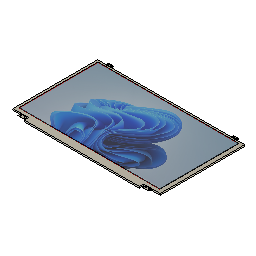
Panel_Enclosure (Autodesk Fusion 360 archive; units mm, degrees)
design "Panel_Physical"
Autodesk Fusion 360 part; units mm, degrees
sketch "Panel_Dims" plane through (0, 0, 0) normal (0, 0, 1) x (1, 0, 0)
  line L0 (-180, 103.5) -> (180, 103.5) construction
  line L1 (180, 103.5) -> (180, -103.5) construction
  line L2 (180, -103.5) -> (-180, -103.5) construction
  line L3 (-180, -103.5) -> (-180, 103.5) construction
  line L4 (0, 0) -> (0, 103.5) construction
  line L5 (0, 0) -> (-180, 0) construction
  line L6 (-160, -103.5) -> (-160, -111.5)
  line L7 (-145, -103.5) -> (-145, -111.5)
  line L8 (-145, -111.5) -> (-160, -111.5)
  line L9 (-142, -103.5) -> (-142, -114)
  line L10 (160, -103.5) -> (160, -111.5)
  line L11 (145, -103.5) -> (145, -111.5)
  line L12 (160, -111.5) -> (145, -111.5)
  line L13 (139.5, -103.5) -> (139.5, -114)
  line L14 (139.5, -114) -> (-142, -114)
  line L15 (-160, 103.5) -> (-160, 109.8)
  line L16 (-160, 109.8) -> (-147, 109.8)
  line L17 (-147, 109.8) -> (-147, 103.5)
  line L18 (160, 103.5) -> (160, 109.8)
  line L19 (160, 109.8) -> (147, 109.8)
  line L20 (147, 109.8) -> (147, 103.5)
  line L21 (-180, 103.5) -> (-180, -103.5)
  line L22 (-180, -103.5) -> (-160, -103.5)
  line L23 (-145, -103.5) -> (-142, -103.5)
  line L24 (145, -103.5) -> (139.5, -103.5)
  line L25 (160, -103.5) -> (180, -103.5)
  line L26 (180, 103.5) -> (180, -103.5)
  line L27 (-160, 103.5) -> (-180, 103.5)
  line L28 (-147, 103.5) -> (147, 103.5)
  line L29 (160, 103.5) -> (180, 103.5)
  line L30 (-142, -103.5) -> (139.5, -103.5)
  circle A0 centre (-156.5, -106.7) radius 1.2
  circle A1 centre (-148.5, -106.7) radius 1.2
  line L31 (-156.5, -106.7) -> (-148.5, -106.7) construction
  circle A2 centre (148.5, -106.7) radius 1.2
  line L32 (148.5, -106.7) -> (156.5, -106.7) construction
  circle A3 centre (156.5, -106.7) radius 1.2
  circle A4 centre (-156.5, 106.7) radius 1.2
  line L33 (-156.5, 106.7) -> (-150.5, 106.7) construction
  circle A5 centre (-150.5, 106.7) radius 1.2
  circle A6 centre (150.5, 106.7) radius 1.2
  line L34 (150.5, 106.7) -> (156.5, 106.7) construction
  circle A7 centre (156.5, 106.7) radius 1.2
  line L35 (-174.55, 99) -> (169.45, 99)
  line L36 (169.45, 99) -> (169.45, -94)
  line L37 (169.45, -94) -> (-174.55, -94)
  line L38 (-174.55, -94) -> (-174.55, 99)
  line L39 (145, -103.5) -> (160, -103.5)
  line L40 (147, 103.5) -> (160, 103.5)
  line L41 (-147, 103.5) -> (-160, 103.5)
  line L42 (-160, -103.5) -> (-145, -103.5)
  line L43 (-73, -103.5) -> (-43, -103.5)
  line L44 (-43, -103.5) -> (-43, -114)
  line L45 (-43, -114) -> (-73, -114)
  line L46 (-73, -114) -> (-73, -103.5)
  line L47 (-45, -105) -> (-70, -105)
  line L48 (-70, -105) -> (-70, -109)
  line L49 (-70, -109) -> (-45, -109)
  line L50 (-45, -109) -> (-45, -105)
  point P0 (-156.5, -106.7)
  dimension "panel_w" = 360
  dimension "panel_h" = 207
  dimension "ear_indent" = 20
  dimension "ear_bottom_w" = 15
  dimension "ear_bottom_h" = 8
  dimension "pcb_left_indent" = 38
  dimension "d37" = 20
  dimension "d40" = 8
  dimension "pcb_chin_h" = 10.5
  dimension "pcb_chin_w" = 281.5
  dimension "d45" = 20
  dimension "ear_top_h" = 6.3
  dimension "ear_top_w" = 13
  dimension "d48" = 20
  dimension "d49" = 6.3
  dimension "d50" = 13
  dimension "hole_dist_x" = 3.5
  dimension "hole_dia" = 2.4
  dimension "hole_dist_y" = 3.2
  dimension "d54" = 2.4
  dimension "hole_bottom_ipd" = 8
  dimension "d62" = 2.4
  dimension "d63" = 2.4
  dimension "d64" = 8
  dimension "d65" = 3.2
  dimension "d66" = 3.5
  dimension "d67" = 2.4
  dimension "d68" = 2.4
  dimension "hole_top_ipd" = 6
  dimension "d70" = 3.5
  dimension "d72" = 3.2
  dimension "d73" = 2.4
  dimension "d74" = 2.4
  dimension "d75" = 6
  dimension "d76" = 3.5
  dimension "d77" = 3.2
  dimension "bezel_left" = 5.45
  dimension "bezel_top" = 4.5
  dimension "active_w" = 344
  dimension "active_h" = 193
  dimension "d98" = 30
  dimension "d99" = 10.5
  dimension "d100" = 137
  dimension "d101" = 25
  dimension "d102" = 4
  dimension "d103" = 5
  dimension "d104" = 2
  constraint horizontal L0
  constraint vertical L1
  constraint horizontal L2
  constraint vertical L3
  constraint coincident L4.start L5.start
  constraint midpoint L0 L4.end
  constraint midpoint L3 L5.end
  constraint horizontal L5
  constraint vertical L4
  constraint coincident L2 L6.start
  constraint perpendicular L2 L6
  constraint coincident L2 L7.start
  constraint perpendicular L2 L7
  constraint coincident L2 L9.start
  constraint perpendicular L2 L9
  constraint coincident L2 L10.start
  constraint perpendicular L2 L10
  constraint equal L6 L7
  constraint coincident L2 L11.start
  constraint perpendicular L2 L11
  constraint equal L10 L11
  constraint equal L8 L12
  constraint coincident L2 L13.start
  constraint perpendicular L2 L13
  constraint equal L9 L13
  constraint perpendicular L9 L14
  constraint coincident L0 L15.start
  constraint perpendicular L0 L15
  constraint perpendicular L3 L16
  constraint coincident L0 L17.end
  constraint perpendicular L0 L17
  constraint coincident L0 L18.start
  constraint perpendicular L0 L18
  constraint perpendicular L18 L19
  constraint coincident L0 L20.end
  constraint perpendicular L0 L20
  constraint coincident P0 A0.centre
  constraint coincident A1.centre L31.end
  constraint horizontal L31
  constraint coincident A2.centre L32.start
  constraint coincident L32.end A3.centre
  constraint horizontal L32
  constraint coincident A4.centre L33.start
  constraint coincident L33.end A5.centre
  constraint horizontal L33
  constraint coincident A6.centre L34.start
  constraint coincident L34.end A7.centre
  constraint horizontal L34
  constraint horizontal L35
  constraint vertical L36
  constraint horizontal L37
  constraint vertical L38
  constraint horizontal L43
  constraint vertical L44
  constraint horizontal L45
  constraint vertical L46
  constraint coincident L30 L43.start
  constraint horizontal L47
  constraint vertical L48
  constraint horizontal L49
  constraint vertical L50
  measures "panel_w" distance of L1.end L2.end
  measures "panel_h" distance of L0.start L2.end
  measures "ear_indent" distance of L2.end L6.start
  measures "ear_bottom_w" distance of L6.start L7.start
  measures "ear_bottom_h" distance of L6.start L6.end
  measures "pcb_left_indent" distance of L2.end L9.start
  measures "d37" distance of L1.end L10
  measures "d40" distance of L10.start L10.end
  measures "pcb_chin_h" distance of L9.start L9.end
  measures "pcb_chin_w" distance of L9.end L13.end
  measures "d45" distance of L0.start L15.start
  measures "ear_top_h" distance of L15.start L15.end
  measures "ear_top_w" distance of L15.end L16.end
  measures "d48" distance of L0.end L18
  measures "d49" distance of L18.start L18.end
  measures "d50" distance of L18.end L19.end
  measures "hole_dist_x" horizontal distance of L6.start P0
  measures "hole_dia" diameter of A0
  measures "hole_dist_y" vertical distance of L6.start P0
  measures "d54" diameter of A1
  measures "hole_bottom_ipd" distance of P0 A1.centre
  measures "d62" diameter of A2
  measures "d63" diameter of A3
  measures "d64" distance of L32.end A2.centre
  measures "d65" distance of L2 L32.end
  measures "d66" distance of L10 L32.end
  measures "d67" diameter of A4
  measures "d68" diameter of A5
  measures "hole_top_ipd" distance of L33.end A4.centre
  measures "d70" distance of L15 A4.centre
  measures "d72" distance of L27 A4.centre
  measures "d73" diameter of A6
  measures "d74" diameter of A7
  measures "d75" distance of L34.end A6.centre
  measures "d76" distance of L18 L34.end
  measures "d77" distance of L0 L34.end
  measures "bezel_left" distance of L3 L38
  measures "bezel_top" distance of L27 L35
  measures "active_w" distance of L35.start L35.end
  measures "active_h" distance of L35.end L36.end
  measures "d98" distance of L43.start L43.end
  measures "d99" distance of L43.end L44.end
  measures "d100" distance of L21 L44
  measures "d101" distance of L47.start L47.end
  measures "d102" distance of L47.start L49.end
  measures "d103" distance of L14 L49
  measures "d104" distance of L44 L49.end
extrude "Extrude2" add sketch "Panel_Dims" against normal blind 3.8 from surface at 3.8 contours L9 L14 L30 L46 | L14 L30 L43 L44 L45 L46 | L13 L14 L30 L44 | L47 L48 L49 L50 makes body 1
extrude "Extrude4" add sketch "Panel_Dims" along normal blind 3 separate body contours L35 L36 L37 L38 makes body 2
extrude "Extrude5" add sketch "Panel_Dims" along normal blind 3.8 contours L21 L22 L23 L24 L25 L26 L27 L28 L29 L30 L39 L40 L41 L42 L43 bodies 1 2
extrude "Extrude6" add sketch "Panel_Dims" along normal blind 0.3 from surface at 3 contours L6 L7 L8 L42 | L15 L16 L17 L41 | L18 L19 L20 L40 | L10 L11 L12 L39 bodies 1
extrude "Extrude7" cut sketch "Panel_Dims" along normal blind 1 contours L47 L48 L49 L50 bodies 1
equation "d37 = ear_indent"
equation "d40 = ear_bottom_h"
equation "d45 = ear_indent"
equation "d48 = ear_indent"
equation "d49 = ear_top_h"
equation "d50 = ear_top_w"
equation "d54 = hole_dia"
equation "d62 = hole_dia"
equation "d63 = hole_dia"
equation "d64 = hole_bottom_ipd"
equation "d65 = hole_dist_y"
equation "d66 = hole_dist_x"
equation "d67 = hole_dia"
equation "d68 = hole_dia"
equation "d70 = hole_dist_x"
equation "d72 = hole_dist_y"
equation "d73 = hole_dia"
equation "d74 = hole_dia"
equation "d75 = hole_top_ipd"
equation "d76 = hole_dist_x"
equation "d77 = hole_dist_y"
equation "pcb_thickness = -3,8 mm"
equation "screen_thicc = panel_thicc - 0,8 mm"
equation "panel_thicc = 3,8 mm"
equation "d94 = screen_thicc"
equation "d97 = panel_thicc"
named bodies: "Panel"
